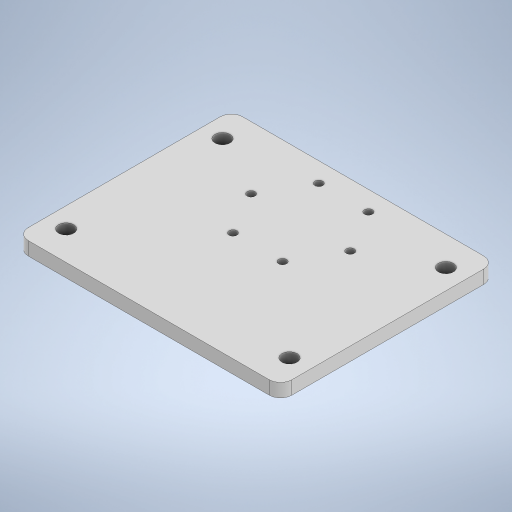
# Autodesk Inventor part: Module_base_Icicles25
Saved by Autodesk Inventor 2023 (Build 270158000, 158)
## iProperties
Created: 2022-10-28
Part Number: Module_base_Icicles25
Material: Generic
Document SubType Name: Modeling
Designer: incep
Density: 1 g/cm^3
Appearance: Default
Author: incep
Autodesk Inventor part; units mm, degrees
ref_plane "YZ Plane" through (0, 0, 0) normal (1, 0, 0) x (0, 1, 0)
ref_plane "XZ Plane" through (0, 0, 0) normal (0, 1, 0) x (-1, 0, 0)
ref_plane "XY Plane" through (0, 0, 0) normal (0, 0, 1) x (1, 0, 0)
sketch "Sketch1" plane through (0, 0, 0) normal (0, 1, 0) x (-1, 0, 0)
  line L0 (54, -48) -> (-54, -48)
  line L1 (-59, -43) -> (-59, 43)
  line L2 (-54, 48) -> (54, 48)
  line L3 (59, 43) -> (59, -43)
  line L4 (50, -35) -> (-50, -35) construction
  line L5 (-50, -35) -> (-50, 35) construction
  line L6 (-50, 35) -> (50, 35) construction
  line L7 (50, 35) -> (50, -35) construction
  arc A0 (59, 43) -> (54, 48) centre (54, 43) ccw
  arc A1 (-54, 48) -> (-59, 43) centre (-54, 43) ccw
  arc A2 (-59, -43) -> (-54, -48) centre (-54, -43) ccw
  arc A3 (54, -48) -> (59, -43) centre (54, -43) ccw
  circle A4 centre (50, -35) radius 3.4
  circle A5 centre (50, 35) radius 3.4
  circle A6 centre (-50, -35) radius 3.4
  circle A7 centre (-50, 35) radius 3.4
  line L8 (0, -20) -> (0, 20) construction
  line L9 (25, -20) -> (25, 20) construction
  line L10 (-25, 20) -> (-25, -20) construction
  arc A8 (-25, -20) -> (25, -20) centre (0, -20) ccw construction
  arc A9 (25, 20) -> (-25, 20) centre (0, 20) ccw construction
  circle A10 centre (0, -20) radius 22.2 construction
  circle A11 centre (-22.2, -20) radius 1.8
  circle A12 centre (-11.1, -39.2258) radius 1.8
  circle A13 centre (11.1, -39.2258) radius 1.8
  circle A14 centre (22.2, -20) radius 1.8
  circle A15 centre (11.1, -0.7742) radius 1.8
  circle A16 centre (-11.1, -0.7742) radius 1.8
  point P0 (0, 0)
  point P1 (-59, 0)
  point P2 (0, -48)
  point P3 (0, -35)
  point P4 (-50, 0)
  point P5 (0, 0)
  dimension "d17" = 44.4
  dimension "d0" = 96
  dimension "d1" = 118
  dimension "d2" = 70
  dimension "d3" = 100
  dimension "d4" = 5
  dimension "d5" = 6.8
  dimension "d6" = 6.8
  dimension "d8" = 6.8
  dimension "d10" = 6.8
  dimension "d13" = 25
  dimension "d14" = 40
  dimension "d23" = 3.6
  dimension "d26" = 360
  constraints: 24 end point, 16 centre point, 12 point on circle, 12 tangent, 6 coincident, 5 midpoint, 5 parallel, 4 horizontal alignment, 3 equal radius, 2 horizontal, 2 perpendicular, 2 vertical alignment, 1 vertical, 15 other
  measures "d0" distance between parallel lines of L2 L0
  measures "d1" distance between parallel lines of L1 L3
  measures "d2" distance between parallel lines of L6 L4
  measures "d3" distance between parallel lines of L7 L5
  measures "d4" radius of A0
  measures "d5" diameter of A4
  measures "d6" diameter of A5
  measures "d8" diameter of A6
  measures "d10" diameter of A7
  measures "d13" radius of A8
  measures "d14" distance of L8.end L8.start
  measures "d23" diameter of A11
extrude "Extrusion1" add sketch "Sketch1" along normal blind 6
equation "\"d17\" = iciclesMountD"
equation "\"d0\" = moduleHeight"
equation "\"d1\" = moduleWidth"
equation "\"d2\" = moduleMountH"
equation "\"d3\" = moduleMountW"
equation "\"d4\" = moduleCornerR"
equation "\"d5\" = moduleMountD"
equation "\"d6\" = moduleMountD"
equation "\"d8\" = moduleMountD"
equation "\"d10\" = moduleMountD"
equation "\"d13\" = moduleOpeningR"
equation "\"d14\" = moduleOpeningH"
equation "\"d23\" = clearanceM3"
equation "\"d15\" = thickness"
equation "\"moduleWidth\" = 118"
equation "\"moduleHeight\" = 96"
equation "\"moduleMountW\" = 100"
equation "\"moduleMountH\" = 70"
equation "\"moduleMountD\" = 6.8"
equation "\"moduleCornerR\" = 5"
equation "\"moduleOpeningR\" = 25"
equation "\"moduleOpeningH\" = 40"
equation "\"thickness\" = 6"
equation "\"insertDrillM3\" = 4"
equation "\"clearanceM6\" = 3.6"
equation "\"d18\" = clearanceM6"
equation "\"d21\" = 360deg"
equation "\"d9\" = iciclesMountD"
equation "\"d22\" = 360deg"
equation "\"d25\" = 0"
equation "\"iciclesPlugD\" = 35.5"
equation "\"chairThickness\" = 12.7"
equation "\"isiclesBaseThickness\" = 3"
equation "\"d29\" = isiclesBaseThickness"
equation "\"isiclesPlugT\" = 7.4"
equation "\"compressedGasket\" = 0.5"
equation "\"d30\" = isiclesPlugT + chairThickness + compressedGasket"
equation "\"d31\" = 0"
equation "\"d33\" = 0"
equation "\"d34\" = isiclesBaseThickness"
equation "\"d35\" = 0"
equation "\"iciclesPlugNeck\" = 16"
equation "\"d38\" = 0"
equation "\"headClearanceM3\" = 5.6"
equation "\"d42\" = 360deg"
equation "\"d45\" = 0"
equation "\"iciclesFilletR\" = 2"
equation "\"d46\" = iciclesFilletR"
equation "\"d47\" = iciclesFilletR"
equation "\"clearanceM3\" = 3.6"
equation "\"icicles25D\" = 36.8"
equation "\"icicles25T\" = 8"
equation "\"icicles25ND\" = 18"
equation "\"insertM3\" = 4"
equation "\"d11\" = insertM3"
equation "\"d36\" = iciclesMountNeckD"
equation "\"d39\" = headClearanceM3"
equation "\"iciclesMountD\" = 44.4"
equation "\"iciclesMountNeckD\" = 19"
body "Solid1"
